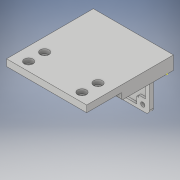
# Autodesk Inventor part: Encoder_Motor_Mount_test
Saved by Autodesk Inventor 2019 (Build 230136000, 136)
## iProperties
Created: 2019-10-02
Part Number: Encoder_Motor_Mount_test
Material: Generic
Document SubType Name: Modeling
Designer: isaac
Density: 1 g/cm^3
Appearance: Default
Author: isaac
Autodesk Inventor part; units mm, degrees
ref_plane "YZ Plane" through (0, 0, 0) normal (1, 0, 0) x (0, 1, 0)
ref_plane "XZ Plane" through (0, 0, 0) normal (0, 1, 0) x (-1, 0, 0)
ref_plane "XY Plane" through (0, 0, 0) normal (0, 0, 1) x (1, 0, 0)
sketch "Sketch1" plane through (0, 0, 0) normal (0, 1, 0) x (-1, 0, 0)
  line L0 (0, 0) -> (60, 0)
  line L1 (60, 0) -> (60, -65)
  line L2 (60, -65) -> (0, -65)
  line L3 (0, -65) -> (0, 0)
  dimension "d0" = 60
  dimension "d1" = 65
  constraints: 8 end point, 2 parallel, 1 horizontal, 1 perpendicular
  measures "d0" distance of L1.end L2.end
  measures "d1" distance of L0.end L1.end
extrude "Extrusion1" add sketch "Sketch1" along normal blind 10
sketch "Sketch2" plane through (0, 10, 0) normal (0, 1, 0) x (1, 0, 0)
  line L0 (-60, 0) -> (0, 0) construction
  line L1 (-60, 0) -> (0, 0) construction
  line L2 (0, 0) -> (0, 25) construction
  line L3 (0, 25) -> (-60, 25) construction
  line L4 (-60, 25) -> (-60, 0) construction
  line L5 (-60, 0) -> (0, 25) construction
  line L6 (0, 0) -> (-60, 25) construction
  line L7 (-50, 6.5) -> (-10, 6.5) construction
  line L8 (-10, 6.5) -> (-10, 18.5) construction
  line L9 (-10, 18.5) -> (-50, 18.5) construction
  line L10 (-50, 18.5) -> (-50, 6.5) construction
  line L11 (-50, 6.5) -> (-10, 18.5) construction
  line L12 (-10, 6.5) -> (-50, 18.5) construction
  point P0 (-30, 12.5)
  dimension "d4" = 60
  dimension "d5" = 25
  dimension "d6" = 40
  dimension "d7" = 12
  constraints: 24 end point, 4 coincident, 4 parallel, 3 midpoint, 2 horizontal, 2 perpendicular
  measures "d4" distance of L3.end L2.end
  measures "d5" distance of L2.end L1.end
  measures "d6" distance of L9.end L8.end
  measures "d7" distance of L8.end L7.end
hole "Hole1" at (-50, 10, -6.5) at (-50, 10, -18.5) at (-10, 10, -18.5) at (-10, 10, -6.5) direction (0, -1, 0) diameter 3.2 end through all counterbore diameter 6.5 counterbore depth 3.25
sketch "Sketch3" plane through (0, 0, 0) normal (0, -1, 0) x (1, 0, 0)
  line L0 (0, 0) -> (-60, 0) projected
  line L1 (0, 0) -> (-60, 0)
  line L2 (-60, 0) -> (-60, -26)
  line L3 (-60, -26) -> (0, -26)
  line L4 (0, -26) -> (0, 0)
  dimension "d15" = 60
  dimension "d16" = 26
  constraints: 8 end point, 2 parallel, 1 horizontal, 1 perpendicular
  measures "d15" distance of L3.end L2.end
  measures "d16" distance of L2.end L1.end
extrude "Extrusion2" cut sketch "Sketch3" against normal blind 5
sketch "Sketch4" plane through (0, 0, 0) normal (0, -1, 0) x (1, 0, 0)
  line L0 (-60, 0) -> (0, 0) construction
  line L1 (-60, -65) -> (-60, 0) construction
  line L2 (0, 0) -> (-60, 0) construction
  line L3 (-60, 0) -> (-60, -57) construction
  line L4 (-60, -57) -> (0, -57) construction
  line L5 (0, -57) -> (0, 0) construction
  line L6 (0, -57) -> (-60, -57) construction
  line L7 (-60, -57) -> (-60, -58.25) construction
  line L8 (-60, -58.25) -> (0, -58.25) construction
  line L9 (0, -58.25) -> (0, -57) construction
  line L10 (0, -58.25) -> (-60, -58.25) construction
  line L11 (-60, -58.25) -> (-60, -60.05) construction
  line L12 (-60, -60.05) -> (0, -60.05) construction
  line L13 (0, -60.05) -> (0, -58.25) construction
  line L14 (-30, -60.05) -> (-30, -65.25) construction
  line L15 (-30, -60.05) -> (-13, -60.05)
  line L16 (-13, -60.05) -> (-13, -63.05)
  line L17 (-13, -63.05) -> (-47, -63.05)
  line L18 (-47, -63.05) -> (-47, -60.05)
  line L19 (-30, -60.05) -> (-47, -60.05)
  dimension "d19" = 57
  dimension "d20" = 1.25
  dimension "d21" = 1.8
  dimension "d22" = 17
  dimension "d23" = 3
  dimension "d24" = 34
  constraints: 36 end point, 8 parallel, 5 perpendicular, 5 point on line, 3 horizontal, 1 midpoint, 1 vertical
  measures "d19" distance of L3.end L2.end
  measures "d20" distance of L7.end L6.end
  measures "d21" distance of L11.end L10.end
  measures "d22" distance of L14.start L15.end
  measures "d23" distance of L15.end L16.end
  measures "d24" distance of L16.end L17.end
extrude "Extrusion3" add sketch "Sketch4" along normal blind 33
sketch "Sketch5" plane through (-47, 0, -60.05) normal (0, 0, 1) x (1, 0, 0)
  line L0 (-13, 0) -> (47, 0) construction
  line L1 (17, 0) -> (17, -16.675) construction
  line L2 (29, -28.675) -> (5, -28.675) construction
  line L3 (5, -28.675) -> (5, -4.675) construction
  line L4 (5, -4.675) -> (29, -4.675) construction
  line L5 (29, -4.675) -> (29, -28.675) construction
  line L6 (29, -28.675) -> (5, -4.675) construction
  line L7 (5, -28.675) -> (29, -4.675) construction
  dimension "d27" = 16.675
  dimension "d28" = 24
  dimension "d29" = 24
  constraints: 14 end point, 4 coincident, 3 midpoint, 2 parallel, 1 horizontal, 1 perpendicular, 1 vertical
  measures "d27" distance of L1.start L1.end
  measures "d28" distance of L3.end L4.end
  measures "d29" distance of L2.end L3.end
hole "Hole2" at (-18, -28.675, -60.05) at (-42, -28.675, -60.05) at (-42, -4.675, -60.05) at (-18, -4.675, -60.05) direction (0, 0, -1) diameter 3.2 end through all
sketch "Sketch6" plane through (-47, 0, -60.05) normal (0, 0, 1) x (1, 0, 0)
  point P0 (47, 0)
sketch "Sketch7" plane through (-47, 0, -60.05) normal (0, 0, 1) x (1, 0, 0)
  line L0 (34, 0) -> (34, -33) construction
  line L1 (0, 0) -> (0, -33) construction
  line L2 (34, -33) -> (0, 0) construction
  line L3 (0, -33) -> (34, 0) construction
  line L4 (26, -25.5) -> (8, -25.5)
  line L5 (8, -25.5) -> (8, -7.5)
  line L6 (8, -7.5) -> (26, -7.5)
  line L7 (26, -7.5) -> (26, -25.5)
  line L8 (26, -25.5) -> (8, -7.5) construction
  line L9 (8, -25.5) -> (26, -7.5) construction
  line L10 (31, -24) -> (3, -24)
  line L11 (3, -24) -> (3, -9)
  line L12 (3, -9) -> (31, -9)
  line L13 (31, -9) -> (31, -24)
  line L14 (31, -24) -> (3, -9) construction
  line L15 (3, -24) -> (31, -9) construction
  line L16 (24.5, -30.5) -> (9.5, -30.5)
  line L17 (9.5, -30.5) -> (9.5, -2.5)
  line L18 (9.5, -2.5) -> (24.5, -2.5)
  line L19 (24.5, -2.5) -> (24.5, -30.5)
  line L20 (24.5, -30.5) -> (9.5, -2.5) construction
  line L21 (9.5, -30.5) -> (24.5, -2.5) construction
  point P0 (47, 0)
  point P1 (17, -16.5)
  dimension "d37" = 18
  dimension "d38" = 18
  dimension "d39" = 28
  dimension "d40" = 15
  dimension "d41" = 15
  dimension "d42" = 28
  constraints: 40 end point, 7 midpoint, 6 parallel, 3 horizontal, 3 perpendicular
  measures "d37" distance of L5.end L6.end
  measures "d38" distance of L4.end L5.end
  measures "d39" distance of L11.end L12.end
  measures "d40" distance of L10.end L11.end
  measures "d41" distance of L17.end L18.end
  measures "d42" distance of L16.end L17.end
extrude "Extrusion4" cut sketch "Sketch7" against normal blind 1.5
fillet "Fillet1" radius 5 2 edges at (-47, 0, -61.55) (-13, 0, -61.55)
fillet "Fillet2" radius 3 2 edges at (-13, -33, -61.55) (-47, -33, -61.55)
fillet "Fillet3" radius 1 1 edges at (-30, 0, -26)
body "Solid1"
